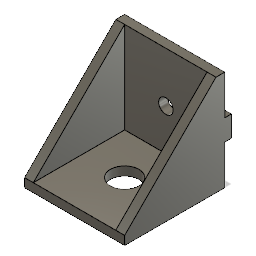
Charger Bracket v3 (Autodesk Fusion 360 design; units mm, degrees)
Autodesk Fusion 360 part; units mm, degrees
note: some values were not read from the file. Set by a fixed rule: which sketch regions a step uses.
sketch "Sketch1" plane through (0, 0, 0) normal (0, 1, 0) x (1, 0, 0)
  line L0 (22.5, 22.5) -> (-22.5, 22.5)
  line L1 (-22.5, 22.5) -> (-22.5, -22.5)
  line L2 (-22.5, -22.5) -> (22.5, -22.5)
  line L3 (22.5, -22.5) -> (22.5, 22.5)
  line L4 (22.5, 22.5) -> (-22.5, -22.5) construction
  line L5 (-22.5, 22.5) -> (22.5, -22.5) construction
  dimension "d1" = 45
  dimension "d2" = 45
  constraint perpendicular L0 L1
  constraint parallel L0 L2
  constraint parallel L1 L3
  constraint horizontal L0
  constraint coincident L4 origin
  constraint coincident L5 origin
  measures "d1" distance of L0.start L2.end L0.end
  measures "d2" distance of L0.start L0.end
extrude "Extrude1" add sketch "Sketch1" along normal blind 4
sketch "Sketch2" plane through (0, 0, -22.5) normal (0, 0, -1) x (-1, 0, 0)
  line L0 (22.5, 0) -> (-22.5, 0)
  line L1 (-22.5, 0) -> (-22.5, 45)
  line L2 (-22.5, 45) -> (22.5, 45)
  line L3 (22.5, 45) -> (22.5, 0)
  point P0 (-22.5, 0)
  point P1 (22.5, 0)
  dimension "d12" = 45
  constraint horizontal L0
  constraint vertical L1
  constraint horizontal L2
  constraint vertical L3
  constraint coincident L0 P0
  constraint coincident L1 P0
  constraint coincident L3 P1
  measures "d12" distance of P0 L1.end
extrude "Extrude4" add sketch "Sketch2" against normal blind 4
sketch "Sketch3" plane through (-22.5, 0, 0) normal (-1, 0, 0) x (0, 0, 1)
  line L0 (-22.5, 0) -> (22.5, 0)
  line L1 (22.5, 0) -> (22.5, 4)
  line L2 (22.5, 4) -> (-18.5, 4)
  line L3 (-22.5, 45) -> (-22.5, 0)
  line L4 (-18.5, 45) -> (-18.5, 4)
  line L5 (22.5, 4) -> (-18.5, 45)
  line L6 (-18.5, 4) -> (-18.5, 45)
  line L7 (-18.5, 45) -> (-22.5, 45)
  constraint coincident L2.end L4.end
  constraint coincident L1.end L2.start
  constraint coincident L4.start L5.end
extrude "Extrude3" add sketch "Sketch3" against normal blind 4 contours L2 L4 L5 L6
mirror "Mirror1" about plane through (0, 0, 0) normal (1, 0, 0) of "Extrude3"
sketch "Sketch6" plane through (0, 0, -22.5) normal (0, 0, -1) x (-1, 0, 0)
  line L0 (-22.5, 0) -> (22.5, 0)
  line L1 (22.5, 0) -> (22.5, 45)
  line L2 (22.5, 45) -> (-22.5, 45)
  line L3 (-22.5, 45) -> (-22.5, 0)
  line L4 (22.5, 27.25) -> (-22.5, 27.25)
  line L5 (-22.5, 27.25) -> (-22.5, 17.75)
  line L6 (-22.5, 17.75) -> (22.5, 17.75)
  line L7 (22.5, 17.75) -> (22.5, 27.25)
  line L8 (22.5, 27.25) -> (-22.5, 17.75) construction
  line L9 (-22.5, 27.25) -> (22.5, 17.75) construction
  line L10 (0, 0) -> (0, 6.5) construction
  line L11 (12.5, 27.25) -> (-12.5, 27.25)
  line L12 (-12.5, 27.25) -> (-12.5, 17.75)
  line L13 (-12.5, 17.75) -> (12.5, 17.75)
  line L14 (12.5, 17.75) -> (12.5, 27.25)
  line L15 (12.5, 27.25) -> (-12.5, 17.75) construction
  line L16 (-12.5, 27.25) -> (12.5, 17.75) construction
  point P0 (0, 22.5)
  point P1 (0, 22.5)
  dimension "d31" = 9.5
  dimension "d32" = 22.5
  dimension "d35" = 25
  constraint perpendicular L4 L5
  constraint parallel L4 L6
  constraint parallel L5 L7
  constraint horizontal L4
  constraint coincident L8 P1
  constraint coincident L9 P1
  constraint coincident L10.start origin
  constraint vertical L10
  constraint coincident P1 L10
  constraint coincident L1.end L7
  constraint perpendicular L11 L12
  constraint parallel L11 L13
  constraint parallel L12 L14
  constraint horizontal L11
  constraint coincident L4 L11.start
  constraint coincident L15 P1
  constraint coincident L16 P1
  constraint coincident P1 P0
  measures "d31" distance of L4 L6
  measures "d32" distance of L10.start P1
  measures "d35" distance of L12 L14
extrude "Extrude7" add sketch "Sketch6" along normal blind 3 contours L3 L4 L5 L6 L12 | L1 L4 L6 L7 L14
sketch "Sketch4" plane through (0, 0, -18.5) normal (0, 0, 1) x (1, 0, 0)
  line L0 (18.5, 45) -> (-18.5, 45)
  line L1 (-18.5, 45) -> (-18.5, 4)
  line L2 (-18.5, 4) -> (18.5, 4)
  line L3 (22.5, 45) -> (-22.5, 45)
  line L4 (-22.5, 0) -> (22.5, 0)
  line L5 (0, 0) -> (0, 20.1593) construction
  circle A0 centre (0, 22.5) radius 3.25
  dimension "d29" = 6.5
  dimension "d30" = 22.5
  constraint coincident L5.start origin
  constraint perpendicular L2 L5
  constraint coincident L5 A0.centre
  measures "d29" diameter of A0
  measures "d30" distance of L5.start A0.centre
extrude "Extrude5" cut sketch "Sketch4" against normal through all
sketch "Sketch5" plane through (0, 0, 0) normal (0, -1, 0) x (1, 0, 0)
  line L0 (22.5, -22.5) -> (22.5, 22.5)
  line L1 (-22.5, 22.5) -> (-22.5, -22.5)
  line L2 (-22.5, -22.5) -> (22.5, -22.5)
  line L3 (-22.5, -22.5) -> (22.5, -22.5)
  circle A0 centre (0, 0) radius 6.4
  dimension "d28" = 12.8
  constraint coincident A0.centre origin
  measures "d28" diameter of A0
extrude "Extrude6" cut sketch "Sketch5" against normal blind 4
equation "d30 = ( 45 / 2 ) * 1 mm"
equation "d32 = ( 45 / 2 ) * 1 mm"
